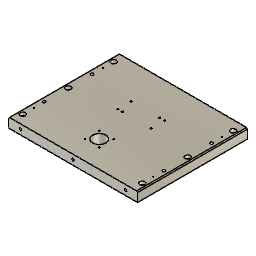
CAD_File 3 (Autodesk Fusion 360 design; units mm, degrees)
Autodesk Fusion 360 part; units mm, degrees
sketch "Sketch3" plane through (0, 0, 0) normal (0, 0, 1) x (1, 0, 0)
  line L0 (135, -115) -> (-135, -115)
  line L1 (-135, -115) -> (-135, 115)
  line L2 (-135, 115) -> (135, 115)
  line L3 (135, 115) -> (135, -115)
  line L4 (135, -115) -> (-135, 115) construction
  line L5 (-135, -115) -> (135, 115) construction
  circle A0 centre (0, -60) radius 14
  circle A1 centre (-15, -45) radius 1.5
  line L6 (0, -25) -> (0, -70) construction
  circle A2 centre (15, -45) radius 1.5
  circle A3 centre (-15, -75) radius 1.5
  circle A4 centre (15, -75) radius 1.5
  line L7 (-182.0885, 0) -> (175, 0) construction
  line L8 (0, 125) -> (0, -125) construction
  dimension "d467" = 28
  dimension "d469" = 3
  dimension "d470" = 15
  dimension "d471" = 15
  dimension "d474" = 60
  dimension "d475" = 115
  dimension "d476" = 135
  dimension "d477" = 15
  dimension "d478" = 15
  dimension "d479" = 15
  dimension "d480" = 15
  constraint horizontal L0
  constraint perpendicular L0 L1
  constraint parallel L0 L2
  constraint parallel L1 L3
  constraint coincident L4 origin
  constraint coincident L5 origin
  constraint vertical L6
  constraint symmetric A1 L6 A2
  constraint perpendicular L3 L7
  constraint vertical L8
  measures "d467" diameter of A0
  measures "d469" diameter of A1
  measures "d470" vertical distance of A0.centre A1.centre
  measures "d471" horizontal distance of A0.centre A1.centre
  measures "d474" distance of A0.centre L7
  measures "d475" distance of L0 L7
  measures "d476" distance of L1 L8
  measures "d477" vertical distance of A0.centre A4.centre
  measures "d478" vertical distance of A0.centre A3.centre
  measures "d479" horizontal distance of A0.centre A3.centre
  measures "d480" horizontal distance of A0.centre A4.centre
extrude "Extrude1" add sketch "Sketch3" against normal blind 20
chamfer "Chamfer1" distance 2 angle 45 2 edges at (-135, 0, 0) (135, 0, 0)
sketch "Sketch4" plane through (0, 0, 0) normal (0, 0, 1) x (-1, 0, 0)
  line L0 (-133, 115) -> (-133, -115)
  line L1 (-133, -115) -> (133, -115)
  line L2 (133, -115) -> (133, 115)
  line L3 (133, 115) -> (-133, 115)
  circle A0 centre (15, 75) radius 1.5
  circle A1 centre (-15, 75) radius 1.5
  circle A2 centre (0, 60) radius 14
  circle A3 centre (15, 45) radius 1.5
  circle A4 centre (-15, 45) radius 1.5
  line L4 (150, 0) -> (-150, 0) construction
  line L5 (0, -130) -> (0, 130) construction
  circle A5 centre (125, -95) radius 3
  circle A6 centre (125, 0) radius 3
  circle A7 centre (125, -50) radius 3
  line L6 (135, -115) -> (135, 115)
  circle A8 centre (125, -95) radius 5.5
  circle A9 centre (125, 0) radius 5.5
  circle A10 centre (-125, -95) radius 5.5
  circle A11 centre (-125, -95) radius 3
  circle A12 centre (-125, -50) radius 3
  circle A13 centre (-125, 0) radius 5.5
  circle A14 centre (-125, 0) radius 3
  circle A15 centre (125, 95) radius 5.5
  circle A16 centre (125, 95) radius 3
  circle A17 centre (125, 50) radius 3
  circle A18 centre (-125, 95) radius 5.5
  circle A19 centre (-125, 95) radius 3
  circle A20 centre (-125, 50) radius 3
  dimension "d536" = 6
  dimension "d537" = 6
  dimension "d538" = 6
  dimension "d539" = 10
  dimension "d540" = 10
  dimension "d541" = 10
  dimension "d542" = 20
  dimension "d543" = 65
  dimension "d544" = 11
  dimension "d545" = 11
  constraint horizontal L4
  constraint perpendicular L3 L5
  constraint coincident L4 A6.centre
  constraint concentric A5 A8
  constraint concentric A6 A9
  constraint symmetric L5 A5 A11
  constraint symmetric L5 A6 A14
  constraint symmetric L5 A7 A12
  constraint symmetric L5 A8 A10
  constraint symmetric L5 A9 A13
  constraint symmetric L4 A5 A16
  constraint symmetric L4 A7 A17
  constraint symmetric L4 A8 A15
  constraint symmetric L4 A10 A18
  constraint symmetric L4 A11 A19
  constraint symmetric L4 A12 A20
  measures "d536" diameter of A5
  measures "d537" diameter of A6
  measures "d538" diameter of A7
  measures "d539" distance of A5.centre L6
  measures "d540" distance of A7.centre L6
  measures "d541" distance of A6.centre L6
  measures "d542" distance of L1 A5.centre
  measures "d543" distance of L1 A7.centre
  measures "d544" diameter of A8
  measures "d545" diameter of A9
extrude "Extrude2" cut sketch "Sketch4" against normal blind 40 contours A5 | A6 | A11 | A14 | A16 | A19
extrude "Extrude3" cut sketch "Sketch4" against normal blind 35 contours A7 | A12 | A17 | A20
extrude "Extrude4" cut sketch "Sketch4" against normal blind 6.5 contours A8 | A9 | A10 | A13 | A15 | A18
sketch "sketch 2210" plane through (0, 135, 0) normal (0, 1, 0) x (-1, 0, 0)
  circle A0 centre (-110, -182.35) radius 3
  circle A1 centre (110, -182.35) radius 3
  circle A2 centre (125, -60) radius 3
  circle A3 centre (0, -10) radius 3
  circle A4 centre (-125, -60) radius 3
  circle A5 centre (-110, -10) radius 3
  circle A6 centre (110, -10) radius 3
  circle A7 centre (125, -132.35) radius 3
  circle A8 centre (0, -182.35) radius 3
  circle A9 centre (-125, -132.35) radius 3
extrude "Extrude5" cut sketch "sketch 2210" against normal blind 40
sketch "sketch 2259" plane through (0, 135, 0) normal (0, 1, 0) x (-1, 0, 0)
  circle A0 centre (-60, -10) radius 3
  circle A1 centre (-60, -182.35) radius 3
  circle A2 centre (60, -182.35) radius 3
  circle A3 centre (60, -10) radius 3
extrude "Extrude6" cut sketch "sketch 2259" against normal blind 35
sketch "sketch 2283" plane through (0, -135, 0) normal (0, -1, 0) x (1, 0, 0)
  circle A0 centre (-110, -182.35) radius 3
  circle A1 centre (110, -182.35) radius 3
  circle A2 centre (125, -60) radius 3
  circle A3 centre (0, -10) radius 3
  circle A4 centre (-125, -60) radius 3
  circle A5 centre (-110, -10) radius 3
  circle A6 centre (110, -10) radius 3
  circle A7 centre (125, -132.35) radius 3
  circle A8 centre (0, -182.35) radius 3
  circle A9 centre (-125, -132.35) radius 3
extrude "Extrude7" cut sketch "sketch 2283" against normal blind 40
thread "Thread1" "ISO Metric profile 6.0 M6x1 6H" major diameter 6.147 minor diameter 5.035 pitch 1 angle 60 resizes the face on face at (-107.0149, -108.3333, -10.2987) on face at (2.9851, -108.3333, -10.2987) on face at (-112.9963, 101.6667, -10.1495) on face at (112.9851, -108.3333, -10.2987) on face at (-2.9963, 101.6667, -10.1495) on face at (107.0149, 108.3333, -10.2987)
sketch "Sketch5" plane through (0, 0, 0) normal (0, 0, 1) x (-1, 0, 0)
  circle A0 centre (-125, 95) radius 5.5
  circle A1 centre (125, -95) radius 5.5
  circle A2 centre (-125, 0) radius 5.5
  circle A3 centre (125, 95) radius 5.5
  circle A4 centre (125, 0) radius 5.5
  circle A5 centre (-125, -95) radius 5.5
  circle A6 centre (125, 50) radius 3
  circle A7 centre (-125, 50) radius 3
  circle A8 centre (125, -50) radius 3
  circle A9 centre (-125, -50) radius 3
  line L0 (-133, 115) -> (-133, -115)
  line L1 (-133, -115) -> (133, -115)
  line L2 (133, -115) -> (133, 115)
  line L3 (133, 115) -> (-133, 115)
  circle A10 centre (15, 75) radius 1.5
  circle A11 centre (-15, 75) radius 1.5
  circle A12 centre (0, 60) radius 14
  circle A13 centre (15, 45) radius 1.5
  circle A14 centre (-15, 45) radius 1.5
  circle A15 centre (125, -72) radius 1.5
  circle A16 centre (125, 72) radius 1.5
  circle A17 centre (-125, 72) radius 1.5
  circle A18 centre (-125, -72) radius 1.5
  circle A19 centre (34.9999, -41.5001) radius 2.1
  circle A20 centre (34.9999, -13.5001) radius 2.1
  circle A21 centre (24.9999, -13.5001) radius 2
  circle A22 centre (-35.0001, -13.5001) radius 2.1
  circle A23 centre (-35.0001, -41.5001) radius 2.1
  circle A24 centre (-25.0001, -41.5001) radius 2
  dimension "d726" = 3
  dimension "d727" = 3
  dimension "d728" = 3
  dimension "d729" = 3
  measures "d726" diameter of A15
  measures "d727" diameter of A16
  measures "d728" diameter of A17
  measures "d729" diameter of A18
extrude "Extrude8" cut sketch "Sketch5" against normal blind 15 contours A19 | A20 | A22 | A23
extrude "Extrude9" cut sketch "Sketch5" against normal blind 10 contours A21 | A24
extrude "Extrude10" cut sketch "Sketch5" against normal blind 10 contours A15 | A16 | A17 | A18
thread "Thread2" "ISO Metric profile 3.0 M3x0.5 6H" major diameter 3.086 minor diameter 2.529 pitch 0.5 angle 60 resizes the face on face at (123.8043, -72.9057, -6.6667) on face at (123.5905, 71.487, -6.6667) on face at (-126.4095, -72.513, -6.6667) on face at (-126.1957, 71.0943, -6.6667)
thread "Thread3" "ISO Metric profile 4.0 M4x0.7 6H" major diameter 4.1095 minor diameter 3.332 pitch 0.7 angle 60 resizes the face on face at (-37.0895, 41.7092, -10) on face at (-37.0895, 13.7092, -10) on face at (32.9105, 41.7092, -10) on face at (32.9105, 13.7092, -10)
sketch "Sketch6" plane through (0, 0, -20) normal (0, 0, -1) x (1, 0, 0)
  circle A0 centre (-125, 50) radius 3
  circle A1 centre (125, 50) radius 3
  circle A2 centre (-125, -50) radius 3
  circle A3 centre (125, -50) radius 3
  circle A4 centre (125, 95) radius 3
  circle A5 centre (-125, -95) radius 3
  circle A6 centre (125, 0) radius 3
  circle A7 centre (-125, 95) radius 3
  circle A8 centre (-125, 0) radius 3
  circle A9 centre (125, -95) radius 3
  circle A10 centre (-15, 75) radius 1.5
  circle A11 centre (15, 75) radius 1.5
  circle A12 centre (0, 60) radius 14
  circle A13 centre (-15, 45) radius 1.5
  circle A14 centre (15, 45) radius 1.5
  line L0 (-135, -115) -> (135, -115)
  line L1 (135, -115) -> (135, 115)
  line L2 (135, 115) -> (-135, 115)
  line L3 (-135, 115) -> (-135, -115)
  line L4 (1.4109, 97.447) -> (0.1831, 97.447)
  line L5 (0.1831, 97.447) -> (0.1831, 105.271)
  spline S0 degree 2 poles (0.1831, 105.271) (-0.2603, 104.8481) (-0.9799, 104.4251) knots 0 0 0 1 1 1
  spline S1 degree 2 poles (-0.9799, 104.4251) (-1.6996, 104.0022) (-2.2726, 103.7908) knots 0 0 0 1 1 1
  line L6 (-2.2726, 103.7908) -> (-2.2726, 104.9777)
  spline S2 degree 2 poles (-2.2726, 104.9777) (-1.2426, 105.462) (-0.4718, 106.1509) knots 0 0 0 1 1 1
  spline S3 degree 2 poles (-0.4718, 106.1509) (0.299, 106.8399) (0.6196, 107.4879) knots 0 0 0 1 1 1
  line L7 (0.6196, 107.4879) -> (1.4109, 107.4879)
  line L8 (1.4109, 107.4879) -> (1.4109, 97.447)
extrude "Extrude11" cut sketch "Sketch6" against normal blind 0.5 contours L4 L5 S0 S1 L6 S2 S3 L7 L8
